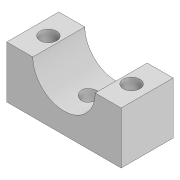
# Autodesk Inventor part: Tube_mount_centering
Saved by Autodesk Inventor 2022 (Build 260153000, 153)
## iProperties
Created: 2022-04-28
Part Number: Tube_mount_centering
Material: Generic
Document SubType Name: Modeling
Designer: dell
Density: 1 g/cm^3
Appearance: Default
Author: dell
Autodesk Inventor part; units mm, degrees
ref_plane "YZ Plane" through (0, 0, 0) normal (1, 0, 0) x (0, 1, 0)
ref_plane "XZ Plane" through (0, 0, 0) normal (0, 1, 0) x (-1, 0, 0)
ref_plane "XY Plane" through (0, 0, 0) normal (0, 0, 1) x (1, 0, 0)
sketch "Sketch2" plane through (0, 0, 0) normal (0, 0, 1) x (1, 0, 0)
  circle A0 centre (0, 0) radius 6
  line L0 (-11, 0) -> (11, 0)
  line L1 (11, 0) -> (11, -10)
  line L2 (11, -10) -> (-11, -10)
  line L3 (-11, -10) -> (-11, 0)
  circle A1 centre (0, 0) radius 9
  point P0 (6, 0)
  point P1 (-6, 0)
  dimension "d0" = 12
  dimension "d1" = 11
  dimension "d2" = 11
  dimension "d3" = 10
  dimension "d4" = 3
  constraints: 8 end point, 2 centre point, 2 parallel, 1 coincident, 1 horizontal, 1 midpoint, 1 perpendicular
  measures "d0" diameter of A0
  measures "d1" distance from line of A0.centre L3
  measures "d2" distance from line of point (0, 0) L1
  measures "d3" distance from line of point (0, 0) L2
  measures "d4" radial gap between concentric circles of A0 A1
extrude "Extrusion1" add sketch "Sketch2" along normal blind 10 contours L0 A1 A0 | L0 L1 L2 L3 A1 picked at (-7.9128, -0.7179)
sketch "Sketch3" plane through (6, 0, 0) normal (0, 1, 0) x (1, 0, 0)
  circle A0 centre (2, -5) radius 1.6
  line L0 (5, 0) -> (5, -10) projected
  line L1 (5, 0) -> (0, 0) projected
  circle A1 centre (-14, -5) radius 1.6
  line L2 (-17, 0) -> (-17, -10) projected
  line L3 (-12, 0) -> (-17, 0) projected
  point P0 (-6, 0)
  dimension "d7" = 3.2
  dimension "d8" = 3
  dimension "d9" = 5
  dimension "d10" = 3.2
  dimension "d11" = 3
  dimension "d12" = 5
  constraints: 2 centre point
  measures "d7" diameter of A0
  measures "d8" distance from line of L0 A0.centre
  measures "d9" distance from line of L1 A0.centre
  measures "d10" diameter of A1
  measures "d11" distance from line of L2 A1.centre
  measures "d12" distance from line of L3 A1.centre
extrude "Extrusion2" cut sketch "Sketch3" against normal blind 10
sketch "Sketch4" plane through (-11, -10, 0) normal (0, -1, 0) x (1, 0, 0)
  circle A0 centre (11, 5) radius 1.6
  line L0 (0, 0) -> (22, 0) projected
  point P0 (11, 0)
  dimension "d15" = 3.2
  dimension "d16" = 5
  constraints: 1 centre point
  measures "d15" diameter of A0
  measures "d16" distance from line of L0 A0.centre
extrude "Extrusion3" cut sketch "Sketch4" against normal blind 10
equation "\"d2\" = d1"
body "Solid1"
